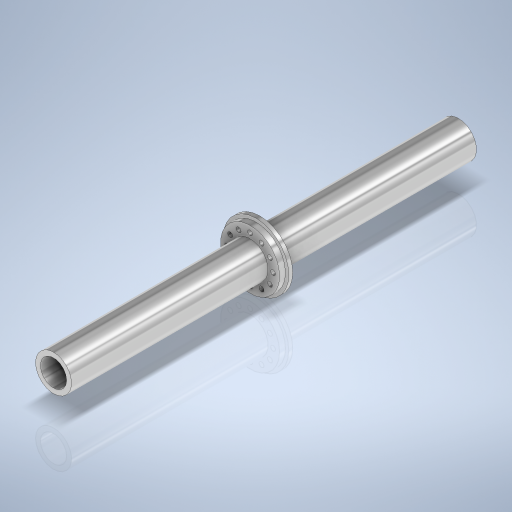
# Autodesk Inventor part: fuel_pipeline
Saved by Autodesk Inventor 2024 (Build 280153000, 153)
## iProperties
Created: 2023-07-07
Part Number: fuel_pipeline
Material: Generic
Document SubType Name: Modeling
Designer: tamiz
Density: 1 g/cm^3
Appearance: Default
Author: tamiz
Autodesk Inventor part; units mm, degrees
ref_plane "YZ Plane" through (0, 0, 0) normal (1, 0, 0) x (0, 1, 0)
ref_plane "XZ Plane" through (0, 0, 0) normal (0, 1, 0) x (-1, 0, 0)
ref_plane "XY Plane" through (0, 0, 0) normal (0, 0, 1) x (1, 0, 0)
sketch "Sketch2" plane through (0, 0, 0) normal (0, 0, 1) x (1, 0, 0)
  circle A0 centre (0, 0) radius 152.4
  circle A1 centre (0, 0) radius 137.16
  circle A2 centre (0, 106.68) radius 11.43
  circle A3 centre (-53.34, 92.3876) radius 11.43
  circle A4 centre (-92.3876, 53.34) radius 11.43
  circle A5 centre (-106.68, 0) radius 11.43
  circle A6 centre (-92.3876, -53.34) radius 11.43
  circle A7 centre (-53.34, -92.3876) radius 11.43
  circle A8 centre (0, -106.68) radius 11.43
  circle A9 centre (53.34, -92.3876) radius 11.43
  circle A10 centre (92.3876, -53.34) radius 11.43
  circle A11 centre (106.68, 0) radius 11.43
  circle A12 centre (92.3876, 53.34) radius 11.43
  circle A13 centre (53.34, 92.3876) radius 11.43
  dimension "d0" = 304.8
  dimension "d1" = 274.32
  dimension "d2" = 22.86
  dimension "d5" = 360
  constraints: 14 centre point, 2 coincident, 25 other
  measures "d0" diameter of A0
  measures "d1" diameter of A1
  measures "d2" diameter of A2
extrude "Extrusion1" add sketch "Sketch2" against normal blind 27.432 contours A1
extrude "Extrusion2" add sketch "Sketch2" against normal blind 18.288 contours A0
sketch "Sketch3" plane through (0, 0, -27.432) normal (0, 0, -1) x (-1, 0, 0)
  circle A0 centre (0, 0) radius 83.82
  dimension "d11" = 167.64
  constraints: 1 centre point, 1 coincident
  measures "d11" diameter of A0
extrude "Extrusion3" add sketch "Sketch3" along normal blind 914.4
sketch "Sketch4" plane through (0, 0, -941.832) normal (0, 0, -1) x (-1, 0, 0)
  circle A0 centre (0, 0) radius 60.96
  dimension "d14" = 121.92
  constraints: 1 centre point, 1 coincident
  measures "d14" diameter of A0
extrude "Extrusion4" cut sketch "Sketch4" against normal blind 1524
mirror "Mirror1" about plane through (0, 0, 0) normal (0, 0, 1) of "Extrusion1", "Extrusion4", "Extrusion3"
body "Solid1"
